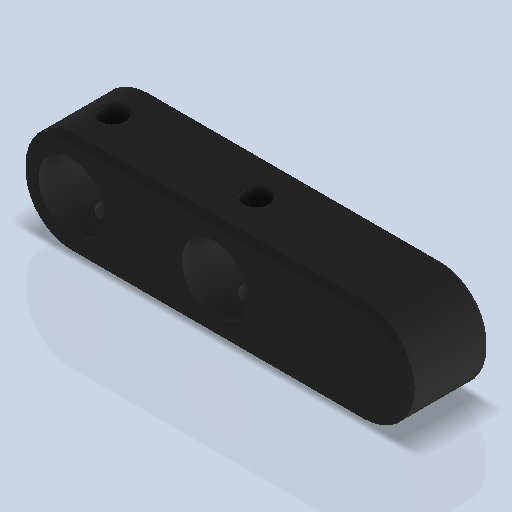
# Autodesk Inventor part: BMS_support
Saved by Autodesk Inventor 2024.2 (Build 282272000, 272)
## iProperties
Created: 2024-05-14
Part Number: BMS_support
Material: Gummi, Silikon
Document SubType Name: Modeling
Designer: Fabri
Density: 1.25 g/cm^3
Appearance: Gummi - Schwarz
Author: Fabri
Autodesk Inventor part; units mm, degrees
ref_plane "YZ Plane" through (0, 0, 0) normal (1, 0, 0) x (0, 1, 0)
ref_plane "XZ Plane" through (0, 0, 0) normal (0, 1, 0) x (-1, 0, 0)
ref_plane "XY Plane" through (0, 0, 0) normal (0, 0, 1) x (1, 0, 0)
sketch "Skizze1" plane through (0, 0, 0) normal (0, 1, 0) x (-1, 0, 0)
  line L0 (14, 5) -> (-14, 5)
  arc A0 (-14, 5) -> (-14, -5) centre (-14, 0) ccw
  line L1 (-14, -5) -> (14, -5)
  arc A1 (14, -5) -> (14, 5) centre (14, 0) ccw
  line L2 (19, 0) -> (-19, 0) construction
  point P0 (0, 0)
  point P1 (0, 0)
  dimension "d0" = 10
  dimension "d1" = 38
  constraints: 6 end point, 6 point on circle, 4 tangent, 2 centre point, 1 coincident, 1 horizontal, 1 horizontal alignment, 1 midpoint, 1 parallel
  measures "d0" distance between parallel lines of L1 L0
  measures "d1" distance of L2.start L2.end
extrude "Extrusion1" add sketch "Skizze1" along normal blind 8
sketch "Skizze3" plane through (0, 8, 0) normal (0, 1, 0) x (1, 0, 0)
  arc A0 (14, -5) -> (14, 5) centre (14, 0) ccw projected
  point P0 (0, 0)
  point P1 (0, 0)
  constraints: 1 coincident
hole "Bohrung2" at (0, 8, 0) direction (0, -1, 0) diameter 6.5 depth 8
chamfer "Fasen1" distance 0.5 angle 45 8 edges at (0, 8, -5) (-19, 8, 0) (0, 8, 5) (19, 8, 0) (0, 0, -5) (-19, 0, 0) (0, 0, 5) (19, 0, 0)
sketch "Skizze2" plane through (0, 8, 0) normal (0, 1, 0) x (1, 0, 0)
  arc A0 (-14, 5) -> (-14, -5) centre (-14, 0) ccw projected
  point P0 (0, 0)
  point P1 (-14, 0)
  constraints: 1 coincident
hole "Bohrung1" at (-14, 8, 0) direction (0, -1, 0) diameter 6.5 depth 8
sketch "Skizze4" plane through (14, 0, -5) normal (0, 0, -1) x (-1, 0, 0)
  line L0 (0, 8) -> (28, 8) projected
  line L1 (0, 0) -> (28, 0) projected
  line L2 (33, 0) -> (33, 8) projected
  line L3 (24.75, 8) -> (31.25, 8) projected
  line L4 (28, 0) -> (28, 8) projected
  point P0 (14, 0)
  point P1 (28, 4)
  point P2 (14, 4)
  point P3 (14, 0)
  point P4 (28, 4)
  dimension "d25" = 4
  constraints: 2 midpoint, 1 coincident, 1 horizontal alignment, 1 vertical alignment
  measures "d25" distance from line of L0 point (28, 4)
hole "Bohrung3" at (-14, 4, -5) at (0, 4, -5) direction (0, 0, 1) diameter 2.5 depth 10
